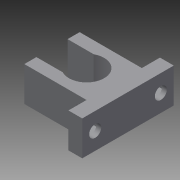
# Autodesk Inventor part: ZAxisEndstopMount
Saved by Autodesk Inventor 2015 SP1 (Build 190203100, 203)
## iProperties
Created: 2015-01-30
Part Number: ZAxisEndstopMount
Material: Generic
Document SubType Name: Modeling
Designer: Jack
Density: 1 g/cm^3
Appearance: Default
Author: Jack
Autodesk Inventor part; units mm, degrees
ref_plane "YZ Plane" through (0, 0, 0) normal (1, 0, 0) x (0, 1, 0)
ref_plane "XZ Plane" through (0, 0, 0) normal (0, 1, 0) x (-1, 0, 0)
ref_plane "XY Plane" through (0, 0, 0) normal (0, 0, 1) x (1, 0, 0)
sketch "Sketch1" plane through (0, 0, 0) normal (0, 0, 1) x (1, 0, 0)
  arc A0 (-2.4, -4.5) -> (-2.4, 4.5) centre (0, 0) ccw
  line L0 (-2.4, 4.5) -> (-10, 4.5)
  line L1 (-10, 4.5) -> (-10, 8)
  line L2 (-10, 8) -> (8, 8)
  line L3 (8, -8) -> (-10, -8)
  line L4 (-10, -8) -> (-10, -4.5)
  line L5 (-10, -4.5) -> (-2.4, -4.5)
  line L6 (8, 8) -> (8, 13.25)
  line L7 (8, -8) -> (8, -13.25)
  line L8 (8, 13.25) -> (12, 13.25)
  line L9 (12, 13.25) -> (12, -13.25)
  line L10 (12, -13.25) -> (8, -13.25)
  dimension "d0" = 10.2
  dimension "d1" = 8
  dimension "d2" = 10
  dimension "d3" = 9
  dimension "d7" = 26.5
  dimension "d8" = 5.25
  dimension "d9" = 4
  dimension "d10" = 8
  constraints: 22 end point, 6 perpendicular, 2 equal length, 2 horizontal, 2 point on circle, 2 point on line, 2 vertical, 1 centre point, 1 coincident, 1 vertical alignment
  measures "d0" diameter of A0
  measures "d1" distance from line of point (0, 0) L3
  measures "d2" distance from line of point (0, 0) L4
  measures "d3" distance between parallel lines of L5 L0
  measures "d7" distance of L8.end L9.end
  measures "d8" distance between parallel lines of L2 L8
  measures "d9" distance of L6.end L8.end
  measures "d10" distance from line of point (0, 0) L6
extrude "Extrusion1" add sketch "Sketch1" along normal blind 10
sketch "Sketch2" plane through (12, -13.25, 0) normal (1, 0, 0) x (0, 0, -1)
  line L0 (0, 0) -> (0, 26.5) projected
  line L1 (0, 26.5) -> (-10, 26.5) projected
  circle A0 centre (-5, 22.75) radius 1.75
  circle A1 centre (-5, 3.75) radius 1.75
  point P0 (0, 13.25)
  dimension "d11" = 3.5
  dimension "d12" = 19
  dimension "d13" = 3.75
  dimension "d14" = 5
  constraints: 2 centre point, 1 equal radius, 1 vertical alignment
  measures "d11" diameter of A0
  measures "d12" distance of A0.centre A1.centre
  measures "d13" distance from line of L1 A0.centre
  measures "d14" distance from line of L0 A0.centre
extrude "Extrusion2" cut sketch "Sketch2" against normal blind 7
sketch "Sketch3" plane through (8, 8, 0) normal (-1, 0, 0) x (0, 0, 1)
  arc A0 (5.9014, 0) -> (4.0986, 0) centre (5, 1.5) ccw projected
  arc A1 (4.0986, -16) -> (5.9014, -16) centre (5, -17.5) ccw projected
  line L0 (1.6514, -17.5) -> (3.3257, -14.6)
  line L1 (3.3257, -14.6) -> (6.6743, -14.6)
  line L2 (6.6743, -14.6) -> (8.3486, -17.5)
  line L3 (8.3486, -17.5) -> (6.6743, -20.4)
  line L4 (6.6743, -20.4) -> (3.3257, -20.4)
  line L5 (3.3257, -20.4) -> (1.6514, -17.5)
  line L6 (1.6514, 1.5) -> (3.3257, 4.4)
  line L7 (3.3257, 4.4) -> (6.6743, 4.4)
  line L8 (6.6743, 4.4) -> (8.3486, 1.5)
  line L9 (8.3486, 1.5) -> (6.6743, -1.4)
  line L10 (6.6743, -1.4) -> (3.3257, -1.4)
  line L11 (3.3257, -1.4) -> (1.6514, 1.5)
  point P0 (0, -8)
  dimension "d17" = 5.8
  constraints: 24 end point, 2 coincident, 2 horizontal, 1 parallel, 26 other
  measures "d17" distance between parallel lines of L1 L4
extrude "Extrusion3" cut sketch "Sketch3" along normal blind 3 and the other way blind 2.6
body "Solid1"
